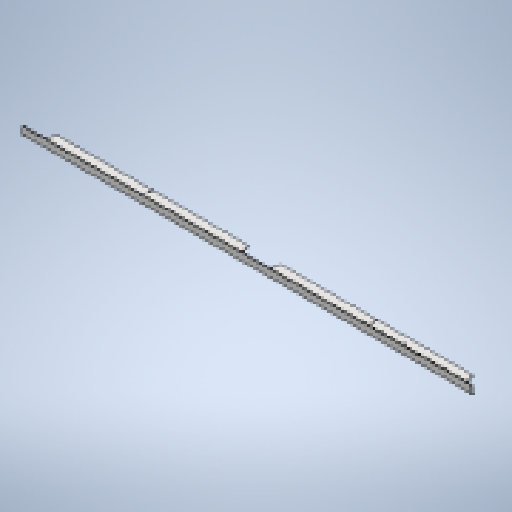
# Autodesk Inventor part: MSC 317 stringer board ##
Saved by Autodesk Inventor 2025 (Build 290162010, 162A)
## iProperties
Created: 2024-04-28
Part Number: MSC 317 stringer board ##
Material: Stainless Steel
Document SubType Name: Sheet Metal
Designer: pokla
Density: 8 g/cm^3
Sheet Metal Rule: AISI304 2mm Die16
Sheet Metal Width: 980,000 mm
Sheet Metal Length: 55,202 mm
Sheet Metal Area: 54097,951 mm^2
Appearance: Default
Stock Number: МОО 317 стрингер борт ##
Flat Pattern Width: 98 cm
Flat Pattern Length: 5.5202 cm
Flat Pattern Area: 540.98 cm^2
Author: admin
Autodesk Inventor part; units mm, degrees
ref_plane "YZ Plane" through (0, 0, 0) normal (1, 0, 0) x (0, 1, 0)
ref_plane "XZ Plane" through (0, 0, 0) normal (0, 1, 0) x (-1, 0, 0)
ref_plane "XY Plane" through (0, 0, 0) normal (0, 0, 1) x (1, 0, 0)
sketch "Sketch1" plane through (0, 0, 0) normal (0, 0, 1) x (1, 0, 0)
  line L0 (-490, 39) -> (490, 39)
  line L1 (490, 39) -> (490, 0)
  line L2 (490, 0) -> (-490, 0)
  line L3 (-490, 0) -> (-490, 39)
  point P0 (0, 0)
  point P1 (0, 0)
  dimension "d0" = 980
  dimension "d1" = 39
  measures "d0" distance of L1.end L2.end
  measures "d1" distance of L0.end L1.end
extrude "Plate1" add sketch "Sketch1" along normal blind 2
sketch "Sketch2" plane through (490, 2, 0) normal (0, -1, 0) x (1, 0, 0)
  line L0 (-980, 0) -> (0, 0)
  line L1 (0, 0) -> (0, 20)
  line L2 (0, 20) -> (-980, 20)
  line L3 (-980, 20) -> (-980, 0)
  constraints: 6 end point, 1 horizontal, 1 perpendicular, 1 vertical
edge flange "Flange1" height 20 angle 90 thickness 2 bend radius 2.75 thickness toward (0, -1, 0) relief round relief width 2 relief depth 1 edges at (0, 0, 2) wall of the first edge with corners at (-490, 2, 0) (490, 2, 0) (490, 2, 20) (-490, 2, 20)
bend "Bend1"
corner "Corner1"
sketch "Sketch9" plane through (0, 0, 2) normal (0, 0, 1) x (1, 0, 0)
  line L0 (-490, 4.75) -> (490, 4.75) projected
  line L1 (490, 39) -> (490, 4.75) projected
  line L2 (-490, 39) -> (490, 39) projected
  line L3 (-490, 4.75) -> (-490, 39) projected
  line L4 (0, 0) -> (0, 39) construction
  circle A0 centre (0, 39) radius 35
  circle A1 centre (490, 39) radius 35
  circle A2 centre (-490, 39) radius 35
  line L5 (246.05, 39) -> (243.95, 39)
  line L6 (243.95, 39) -> (243.95, 29)
  line L7 (243.95, 29) -> (246.05, 29)
  line L8 (246.05, 29) -> (246.05, 39)
  line L9 (-490, 39) -> (490, 39) projected
  line L10 (-246.05, 39) -> (-243.95, 39)
  line L11 (-243.95, 39) -> (-243.95, 29)
  line L12 (-243.95, 29) -> (-246.05, 29)
  line L13 (-246.05, 29) -> (-246.05, 39)
  line L14 (-490, 0) -> (490, 0) projected
  point P0 (-245, 29)
  point P1 (245, 29)
  point P2 (7.2068, 4.75)
  point P3 (35, 39)
  point P4 (-35, 39)
  point P5 (-7.2068, 4.75)
  point P6 (455, 39)
  point P7 (482.7932, 4.75)
  point P8 (-482.7932, 4.75)
  point P9 (-455, 39)
  dimension "d41" = 70
  dimension "d42" = 490
  dimension "d43" = 2.1
  dimension "d44" = 29
  dimension "d45" = 10
  constraints: 18 end point, 4 parallel, 3 centre point, 3 coincident, 3 midpoint, 2 equal radius, 2 horizontal, 2 perpendicular, 2 point on line, 1 collinear, 1 symmetric about line
  measures "d41" diameter of A0
  measures "d42" distance of point (-245, 29) point (245, 29)
  measures "d43" distance of L6.end L7.end
  measures "d44" distance between parallel lines of L14 L7
  measures "d45" distance between parallel lines of L2 L7
extrude "Extrusion4" cut sketch "Sketch9" along normal through all both and the other way through all contours L3 L2 A2 L0 | A0 L2 L0 | L2 L11 L12 L13 | A1 L2 L1 L0 | L2 L8 L7 L6 picked at (-466.9666, 36.3717) picked at (477.9174, 19.2147)
sketch "Sketch10" plane through (0, 0, 2) normal (0, 0, 1) x (1, 0, 0)
  line L0 (425.1819, 23.5318) -> (425.1819, 11.5318) construction
  line L1 (425.1819, 11.5318) -> (225.1819, 11.5318) construction
  line L2 (225.1819, 11.5318) -> (225.1819, 23.5318) construction
  line L3 (225.1819, 23.5318) -> (425.1819, 23.5318) construction
  point P0 (0, 0)
  dimension "d48" = 200
  dimension "d49" = 12
  constraints: 1 horizontal, 2 other
  measures "d48" distance of L0.end L1.end
  measures "d49" distance of L1.end L2.end
mark "Mark2"
equation "\"d1\" = БОРТ_стрингер_4_высота"
equation "\"d2\" = Thickness"
equation "\"d3\" = BendReliefWidth"
equation "\"d4\" = BendReliefDepth"
equation "\"d5\" = MinimumRemnant"
equation "\"d6\" = TransitionRadius"
equation "\"d9\" = BendRadius"
equation "\"d10\" = CornerReliefSize"
equation "\"d11\" = GapSize"
equation "\"d12\" = JacobiRadiusSize"
equation "\"GapSize\" = Thickness"
equation "\"MinimumRemnant\" = 2 * Thickness"
equation "\"BendReliefDepth\" = 0.5 * Thickness"
equation "\"BendReliefWidth\" = Thickness"
equation "\"CornerReliefSize\" = 4 * Thickness"
equation "\"JacobiRadiusSize\" = BendRadius"
equation "\"TransitionRadius\" = BendRadius"
equation "\"БОРТ_стрингер_4_высота\" = 39"
equation "\"Thickness\" = 2"
equation "\"BendRadius\" = 2.75"
body "Solid1"
